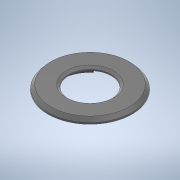
# Autodesk Inventor part: mirror_lock_v4
Saved by Autodesk Inventor 2020 (Build 240168000, 168)
## iProperties
Created: 2024-03-24
Part Number: mirror_lock_v4
Material: Типовые
Document SubType Name: Modeling
Designer: 4s
Density: 1 g/cm^3
Appearance: Гладкая — черная
Mass: 9.10734 g
Surface Area: 89.2393 cm^2
Volume: 9.10734 cm^3
Author: 4s
Autodesk Inventor part; units mm, degrees
ref_plane "YZ Plane" through (0, 0, 0) normal (1, 0, 0) x (0, 1, 0)
ref_plane "XZ Plane" through (0, 0, 0) normal (0, 1, 0) x (-1, 0, 0)
ref_plane "XY Plane" through (0, 0, 0) normal (0, 0, 1) x (1, 0, 0)
sketch "Эскиз1" plane through (0, 0, 0) normal (1, 0, 0) x (0, 1, 0)
  line L0 (0, 0) -> (10.521985, 0) construction
  line L1 (0, 0) -> (0, -19) construction
  line L2 (0, 0) -> (0, -27.3) construction
  line L3 (0, -19) -> (3, -19)
  line L4 (3, -19) -> (3, -27.3)
  line L5 (3, -27.3) -> (0, -27.3)
  line L6 (0, -27.3) -> (0, -19)
  dimension "d0" = 19
  dimension "d1" = 27.3
  dimension "d2" = 3
  constraints: 14 end point, 2 horizontal, 2 parallel, 2 point on line, 1 perpendicular, 1 vertical
  measures "d0" distance of L0.start L1.end
  measures "d1" distance of L0.start L2.end
  measures "d2" distance of L4.end L5.end
sketch "Эскиз1 outline for Вращение1" plane through (0, 0, 0) normal (1, 0, 0) x (0, 1, 0)
  line L0 (0, -19) -> (0, -27.3)
  line L1 (3, -19) -> (0, -19)
  line L2 (3, -27.3) -> (3, -19)
  line L3 (0, -27.3) -> (3, -27.3)
revolve "Вращение1" add sketch "Эскиз1 outline for Вращение1" angle 360 about axis through (0, 0, 0) along (0, 1, 0)
chamfer "Фаска1" distance 2 angle 45 1 edges at (0, 3, 19) measured on face at (2.1778, 3, -24.2689)
chamfer "Фаска2" distance 2 angle 45 1 edges at (0, 3, 27.3) measured on face at (3.853, 3, -24.7322)
sketch "Эскиз2" plane through (0, 0, 0) normal (1, 0, 0) x (0, 1, 0)
  line L0 (0, 0) -> (7.707891, 0) construction
  line L1 (0, 0) -> (0, -24.8) construction
  line L2 (0, 27.3) -> (0, -27.3) construction
  line L3 (0, -25.2) -> (-3.881966, -25.2)
  line L4 (0, -27.3) -> (-3.849721, -27.3)
  line L5 (-4.017311, -25.2) -> (-4.017311, -26.85) construction
  line L6 (0, -25.2) -> (0, -27.3)
  line L7 (-5.878978, 0.249986) -> (-5.878978, -25) construction
  line L8 (-5.878978, -25) -> (-6.121022, -25) construction
  arc A0 (-4.254644, -25.033333) -> (-5.588107, -26.508783) centre (-5, -25.7) ccw
  line L9 (-6, -25) -> (-6, 0) construction
  line L10 (-5.878978, -24.7) -> (-6, -24.7) construction
  line L11 (-4.017311, -25.2) -> (-4.133975, -25.2) construction
  arc A1 (-4.017311, -25.885263) -> (-4.133975, -25.2) centre (-5, -25.7) ccw construction
  arc A2 (-4.254644, -25.033333) -> (-3.881966, -25.2) centre (-3.881966, -24.7) ccw
  line L12 (-5.025935, -26.917567) -> (-5.588107, -26.508783)
  arc A3 (-5.588107, -26.508783) -> (-4.017311, -25.885263) centre (-5, -25.7) ccw construction
  arc A4 (-5.025935, -26.917567) -> (-3.849721, -27.3) centre (-3.849721, -25.3) ccw
  point P0 (-4.285857, -25)
  point P1 (-4.5, -27.3)
  dimension "d10" = 24.8
  dimension "d11" = 4.01731
  dimension "d12" = 0.4
  dimension "d14" = 5.87898
  dimension "d15" = 2
  dimension "d16" = 0.12102
  dimension "d17" = 0.3
  dimension "d18" = 0.5
  dimension "d19" = 50
  dimension "d21" = 4.5
  dimension "d22" = 2
  dimension "d33" = 5
  constraints: 24 end point, 13 point on circle, 10 point on line, 10 tangent, 6 horizontal, 5 centre point, 3 vertical, 1 collinear, 1 midpoint
  measures "d10" distance of L0.start L1.end
  measures "d11" distance of L3.start L5.start
  measures "d12" distance from line of L1.end L3
  measures "d14" distance between parallel lines of L1 L7
  measures "d15" diameter of A0
  measures "d16" distance between parallel lines of L7 L9
  measures "d17" distance from line of point (-4.286, -25) L10
  measures "d18" radius of A2
  measures "d19" diameter of L8 L0
  measures "d21" distance of L2.end point (-4.5, -27.3)
  measures "d22" radius of A4
  measures "d33" distance from line of L6 A0.centre
sketch "Эскиз2 outline for Вращение2" plane through (0, 0, 0) normal (1, 0, 0) x (0, 1, 0)
  arc A0 (-4.254644, -25.033333) -> (-5.588107, -26.508783) centre (-5, -25.7) ccw
  arc A1 (-3.881966, -25.2) -> (-4.254644, -25.033333) centre (-3.881966, -24.7) cw
  line L0 (0, -25.2) -> (-3.881966, -25.2)
  line L1 (0, -27.3) -> (0, -25.2)
  line L2 (-3.849721, -27.3) -> (0, -27.3)
  arc A2 (-5.025935, -26.917567) -> (-3.849721, -27.3) centre (-3.849721, -25.3) ccw
  line L3 (-5.588107, -26.508783) -> (-5.025935, -26.917567)
revolve "Вращение2" add sketch "Эскиз2 outline for Вращение2" angle 50 about axis through (0, 0, 0) along (0, -1, 0)
pattern_circular "Круговой массив1" count 4 over 360 about axis through (0, 1.5, 0) along (0, -1, 0) of "Вращение2"
sketch "Эскиз3" plane through (0, 3, 0) normal (0, 1, 0) x (1, 0, 0)
  circle A0 centre (0, 0) radius 21 construction
  circle A1 centre (0, 0) radius 25.3
  circle A2 centre (0, 0) radius 19 construction
  circle A3 centre (0, 0) radius 21 construction
  arc A4 (-17.039517, 20.306906) -> (-26.508783, 0) centre (0, 0) ccw construction
  circle A5 centre (0, 0) radius 27.3 construction
  circle A6 centre (0, 0) radius 25.3 construction
  circle A7 centre (0, 0) radius 27.3 construction
  circle A8 centre (0, 0) radius 32.5
  dimension "d27" = 65
  constraints: 1 centre point, 1 coincident
  measures "d27" diameter of A8
sketch "Эскиз3 outline for Выдавливание1" plane through (0, 3, 0) normal (0, 1, 0) x (1, 0, 0)
  circle A0 centre (0, 0) radius 32.5
  circle A1 centre (0, 0) radius 25.3
extrude "Выдавливание1" add sketch "Эскиз3 outline for Выдавливание1" against normal blind 2
sketch "Эскиз4" plane through (0, 0, -27.3) normal (0, -1, 0) x (1, 0, 0)
  circle A0 centre (0, 27.3) radius 25.2
  circle A1 centre (0, 27.3) radius 32.5 construction
  circle A2 centre (0, 27.3) radius 27.3 projected
  dimension "d30" = 50.4
  constraints: 1 centre point, 1 coincident
  measures "d30" diameter of A0
sketch "Эскиз4 outline for Выдавливание2" plane through (0, 0, -27.3) normal (0, -1, 0) x (1, 0, 0)
  circle A0 centre (0, 27.3) radius 27.3
  circle A1 centre (0, 27.3) radius 25.2
extrude "Выдавливание2" add sketch "Эскиз4 outline for Выдавливание2" along normal blind 1.5
sketch "Эскиз5" plane through (0, 0, 0) normal (1, 0, 0) x (0, 1, 0)
  line L0 (1, 32.5) -> (1, -32.5) construction
  line L1 (3, -32.5) -> (3, 32.5) construction
  line L2 (-3.881966, 25.2) -> (0, 25.2) construction
  line L3 (1, -27.3) -> (1, 27.3) construction
  line L4 (-3.849721, -20.913013) -> (-1.5, -20.913013) construction
  line L5 (-3.849721, 0) -> (-3.849721, -20.913013) construction
  line L6 (-3.849721, 0) -> (-1.5, 0) construction
  line L7 (-1.5, 17.548102) -> (-1.5, 0) construction
  line L8 (-3.849721, 17.548102) -> (-1.5, 17.548102) construction
  line L9 (-3.849721, 27.3) -> (-3.849721, 17.548102) construction
  line L10 (-3.849721, 27.3) -> (-1.5, 27.3) construction
  line L11 (-1.5, 20.913013) -> (-1.5, 27.3) construction
  line L12 (-3.849721, 20.913013) -> (-1.5, 20.913013) construction
  line L13 (-3.849721, 0) -> (-3.849721, 20.913013) construction
  line L14 (-3.849721, 0) -> (-1.5, 0) construction
  line L15 (-1.5, -17.548102) -> (-1.5, 0) construction
  line L16 (-3.849721, -17.548102) -> (-1.5, -17.548102) construction
  line L17 (-3.849721, -27.3) -> (-3.849721, -17.548102) construction
  line L18 (-3.849721, -27.3) -> (-1.5, -27.3) construction
  line L19 (-1.5, -20.913013) -> (-1.5, -27.3) construction
  line L20 (-4.655238, 37.5) -> (4.442255, 37.5) construction
  line L21 (-1.5, 37.5) -> (-1.5, 36.1)
  line L22 (-1.5, 37.5) -> (-0.1, 37.5)
  line L23 (-0.1, 37.5) -> (3, 34.898791)
  line L24 (3, 34.898791) -> (3, 32.5)
  line L25 (3, 32.5) -> (1, 32.5) construction
  line L26 (-1.5, 36.1) -> (1, 34.002251)
  line L27 (1, 34.002251) -> (1, 32.5)
  line L28 (1, 32.5) -> (1, -32.5)
  line L29 (1, 32.5) -> (3, 32.5)
  point P0 (0, 0)
  dimension "d34" = 37.5
  dimension "d35" = 1.4
  dimension "d36" = 1.4
  dimension "d37" = 40
  constraints: 16 end point, 3 point on line, 2 collinear, 2 horizontal, 2 vertical, 1 parallel, 1 perpendicular
  measures "d34" distance between parallel lines of L20 L6
  measures "d35" distance of L21.start L21.end
  measures "d36" distance of L21.start L22.end
  measures "d37" angle of L20 L23
sketch "Эскиз5 outline for Вращение3" plane through (0, 0, 0) normal (1, 0, 0) x (0, 1, 0)
  line L0 (-1.5, 37.5) -> (-1.5, 36.1)
  line L1 (-0.1, 37.5) -> (-1.5, 37.5)
  line L2 (3, 34.898791) -> (-0.1, 37.5)
  line L3 (3, 32.5) -> (3, 34.898791)
  line L4 (1, 32.5) -> (3, 32.5)
  line L5 (1, 34.002251) -> (1, 32.5)
  line L6 (-1.5, 36.1) -> (1, 34.002251)
revolve "Вращение3" add sketch "Эскиз5 outline for Вращение3" angle 360 about axis through (0, -3.849721, 0) along (0, 1, 0)
